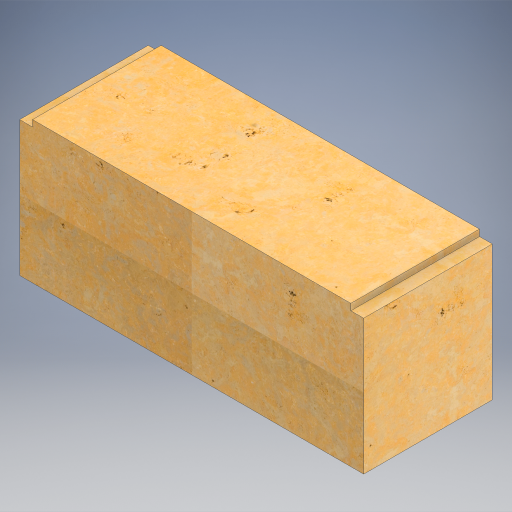
# Autodesk Inventor part: Seat block B
Saved by Autodesk Inventor 2023 (Build 270158030, 158C)
## iProperties
RuleStatus: InUse
Created: 2022-09-14
Part Number: Seat block B
Material: Granite, Cut, Polished
Document SubType Name: Modeling
Designer: awelt
Mass: 1.03776e+06 g
Surface Area: 34751 cm^2
Volume: 384357 cm^3
Density: 2.7 g/cm^3
Appearance: Amber Select
AfterDocSave0: Convert in3 volume to ft3
in3 to ft3: 0.01
TEST: 0.008
Author: awelt
Autodesk Inventor part; units mm, degrees
ref_plane "YZ Plane" through (0, 0, 0) normal (1, 0, 0) x (0, 1, 0)
ref_plane "XZ Plane" through (0, 0, 0) normal (0, 1, 0) x (-1, 0, 0)
ref_plane "XY Plane" through (0, 0, 0) normal (0, 0, 1) x (1, 0, 0)
sketch "Sketch1" plane through (0, 0, 0) normal (0, 0, 1) x (1, 0, 0)
  line L0 (0, 0) -> (1358.9, 0)
  line L1 (1358.9, 0) -> (1358.9, 533.4)
  line L2 (1358.9, 558.8) -> (1308.1, 558.8) construction
  line L3 (0, 558.8) -> (0, 533.4) construction
  line L4 (0, 533.4) -> (50.8, 533.4)
  line L5 (50.8, 533.4) -> (50.8, 558.8)
  line L6 (50.8, 558.8) -> (0, 558.8) construction
  line L7 (0, 533.4) -> (0, 0)
  line L8 (1358.9, 533.4) -> (1308.1, 533.4)
  line L9 (1308.1, 533.4) -> (1308.1, 558.8)
  line L10 (1308.1, 558.8) -> (50.8, 558.8)
  line L11 (1358.9, 533.4) -> (1358.9, 558.8) construction
  dimension "d0" = 1358.9
  dimension "d1" = 558.8
  dimension "d2" = 25.4
  dimension "d3" = 50.8
  dimension "d4" = 25.4
  dimension "d5" = 50.8
  constraints: 24 end point, 7 parallel, 6 perpendicular, 3 horizontal
  measures "d0" distance of L3.start L2.start
  measures "d1" distance of L2.start L0.end
  measures "d2" distance of L4.end L5.end
  measures "d3" distance of L3.end L4.end
  measures "d4" distance of L8.end L2.end
  measures "d5" distance of L1.end L8.end
extrude "Extrusion1" add sketch "Sketch1" along normal blind 508
sketch "Sketch2" plane through (0, 0, 0) normal (0, -1, 0) x (1, 0, 0)
  line L0 (0, 0) -> (0, 508) projected
  line L1 (0, 254) -> (1358.9, 254) construction
  line L2 (1358.9, 0) -> (1358.9, 508) construction
  circle A0 centre (228.6, 254) radius 12.7
  circle A1 centre (1130.3, 254) radius 12.7
  dimension "d8" = 25.4
  dimension "d9" = 25.4
  dimension "d10" = 228.6
  dimension "d11" = 228.6
  constraints: 2 centre point, 2 end point, 2 midpoint, 2 point on line
  measures "d8" diameter of A0
  measures "d9" diameter of A1
  measures "d10" distance from line of L0 A0.centre
  measures "d11" distance from line of A1.centre L2
extrude "Extrusion2" cut sketch "Sketch2" against normal blind 82.55
equation "\"d11\" = d10"
body "Solid1"
